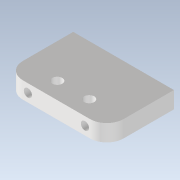
# Autodesk Inventor part: Z-Endstophalter1
Saved by Autodesk Inventor 2022.2 (Build 262287000, 287)
## iProperties
Created: 2021-04-27
Part Number: Z-Endstophalter1
Material: Generic
Document SubType Name: Modeling
Designer: Fabijan_Sven
Density: 1 g/cm^3
Appearance: Default
Author: Fabijan_Sven
Autodesk Inventor part; units mm, degrees
ref_plane "YZ Plane" through (0, 0, 0) normal (1, 0, 0) x (0, 1, 0)
ref_plane "XZ Plane" through (0, 0, 0) normal (0, 1, 0) x (-1, 0, 0)
ref_plane "XY Plane" through (0, 0, 0) normal (0, 0, 1) x (1, 0, 0)
sketch "Sketch1" plane through (0, 0, 0) normal (0, 0, 1) x (1, 0, 0)
  line L0 (-29, 60) -> (29, 60) projected
  line L1 (15, 60) -> (-15, 60)
  line L2 (-15, 60) -> (-15, 55)
  line L3 (-15, 55) -> (15, 55)
  line L4 (15, 55) -> (15, 60)
  point P0 (0, 0)
  point P1 (-15, 60)
  dimension "d0" = 5
  dimension "d1" = 15
  dimension "d2" = 15
  constraints: 8 end point, 2 parallel, 1 horizontal, 1 perpendicular, 1 point on line
  measures "d0" distance of L3.end L1.start
  measures "d1" distance from line of L2 point (0, 0)
  measures "d2" distance from line of L4 point (0, 0)
extrude "Extrusion1" add sketch "Sketch1" along normal blind 20
sketch "Sketch2" plane through (-15, 60, 0) normal (0, 1, 0) x (1, 0, 0)
  circle A0 centre (19.75, -15) radius 1.5
  circle A1 centre (10.25, -15) radius 1.5
  line L0 (30, -20) -> (0, -20) projected
  line L1 (0, 0) -> (0, -20) projected
  point P0 (15, 0)
  dimension "d5" = 9.5
  dimension "d6" = 5
  dimension "d7" = 5
  dimension "d8" = 10.25
  dimension "d9" = 3
  dimension "d10" = 3
  constraints: 2 centre point
  measures "d5" distance of A1.centre A0.centre
  measures "d6" distance from line of A1.centre L0
  measures "d7" distance from line of L0 A0.centre
  measures "d8" distance from line of L1 A1.centre
  measures "d9" diameter of A0
  measures "d10" diameter of A1
hole "Hole1" at (4.75, 60, 15) at (-4.75, 60, 15) direction (0, -1, 0) diameter 3 depth 20 tip angle 118
fillet "Fillet1" radius 5 2 edges at (15, 57.5, 20) (-15, 57.5, 20)
sketch "Sketch3" plane through (0, 0, 0) normal (0, 0, -1) x (-1, 0, 0)
  circle A0 centre (-8.5, 57.5001) radius 1.5 projected
  circle A1 centre (8.5, 57.5) radius 1.5 projected
  point P0 (0, 0)
hole "Hole2" at (8.5, 57.5001, 0) at (-8.5, 57.5, 0) direction (0, 0, 1) diameter 2.459 depth 20 tip angle 118 thread size "M3x0.5" class "6H" standard "ISO Metric profile"
equation "\"d11\" = d10"
body "Solid1"
